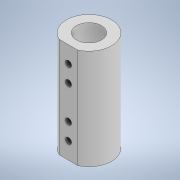
# Autodesk Inventor part: rotaryconnector
Saved by Autodesk Inventor 2020 (Build 240168000, 168)
## iProperties
Created: 2019-06-26
Part Number: rotaryconnector
Material: Generic
Document SubType Name: Modeling
Designer: ColinP
Density: 1 g/cm^3
Appearance: Default
Author: ColinP
Autodesk Inventor part; units mm, degrees
ref_plane "YZ Plane" through (0, 0, 0) normal (1, 0, 0) x (0, 1, 0)
ref_plane "XZ Plane" through (0, 0, 0) normal (0, 1, 0) x (-1, 0, 0)
ref_plane "XY Plane" through (0, 0, 0) normal (0, 0, 1) x (1, 0, 0)
sketch "Sketch10" plane through (0, 0, 0) normal (0, 1, 0) x (-1, 0, 0)
  circle A0 centre (0, 0) radius 3.175
  circle A1 centre (0, 0) radius 5.715
  line L0 (0, 3.175) -> (0, 5.207)
  line L1 (0, 5.207) -> (2.3555, 5.207)
  line L2 (-2.3555, 5.207) -> (0, 5.207)
  dimension "d61" = 6.35
  dimension "d62" = 11.43
  dimension "d63" = 2.032
  constraints: 6 end point, 2 coincident, 2 point on circle, 1 centre point, 1 collinear, 1 perpendicular, 1 point on line, 1 vertical, 1 vertical alignment, 2 other
  measures "d62" diameter of A1
  measures "d63" distance of L0.start L0.end
extrude "Extrusion7" add sketch "Sketch10" along normal blind 25.4 contours A1 L2 L1 picked at (-1.045, 4.4973)
sketch "Sketch12" plane through (-2.3555, 0, 5.207) normal (0, 0, 1) x (1, 0, 0)
  line L0 (2.3555, 0) -> (2.3555, 4.2418)
  line L1 (2.3555, 4.2418) -> (2.3555, 8.4836)
  line L2 (8.0705, 25.4) -> (-3.3595, 25.4) projected
  line L3 (2.3555, 25.4) -> (2.3555, 21.1582)
  line L4 (2.3555, 21.1582) -> (2.3555, 16.9164)
  point P0 (4.711, 25.4)
  point P1 (0, 25.4)
  dimension "d66" = 4.2418
  dimension "d67" = 4.2418
  dimension "d68" = 4.2418
  dimension "d69" = 4.2418
  constraints: 8 end point, 2 point on line, 2 vertical, 1 midpoint
  measures "d66" distance of L0.start L0.end
  measures "d67" distance of L0.end L1.end
  measures "d68" distance of L3.start L3.end
  measures "d69" distance of L3.end L4.end
hole "Hole5" at (0, 21.1582, 5.207) at (0, 16.9164, 5.207) at (0, 8.4836, 5.207) at (0, 4.2418, 5.207) direction (0, 0, -1) diameter 1.567 depth 6.2992 thread size "M2x0.4" class "6H" standard "ISO Metric profile"
body "Solid3"
